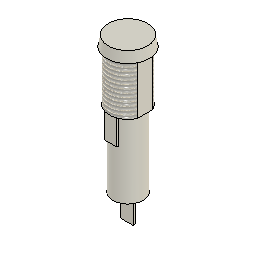
fuse holder 15A v2 (Autodesk Fusion 360 design; units mm, degrees)
Autodesk Fusion 360 part; units mm, degrees
note: some values were not read from the file. Set by a fixed rule: which face or edge a step refers to.
sketch "Sketch1" plane through (0, 0, 0) normal (0, 1, 0) x (1, 0, 0)
  line L0 (0, -54.2) -> (7.7947, -54.2)
  line L1 (7.7947, -54.2) -> (8.5, -50.2)
  line L2 (8.5, -50.2) -> (7.6, -50.2)
  line L3 (7.6, -50.2) -> (7.6, -30.2)
  line L4 (7.6, -30.2) -> (6, -30.2)
  line L5 (6, -30.2) -> (6, 0)
  line L6 (6, 0) -> (0, 0)
  line L7 (0, -54.2) -> (0, 0)
  dimension "d1" = 8.5
  dimension "d2" = 4
  dimension "d3" = 100
  dimension "d4" = 54.2
  dimension "d5" = 15.2
  dimension "d6" = 20
  dimension "d7" = 6
  constraint horizontal L0
  constraint parallel L0 L2
  constraint perpendicular L2 L3
  constraint perpendicular L3 L4
  constraint perpendicular L4 L5
  constraint perpendicular L5 L6
  constraint perpendicular L6 L7
  constraint coincident L6.end L7
  constraint coincident L6.end L7.end
  measures "d1" horizontal distance of L6.end L1.end
  measures "d2" vertical distance of L0.end L1.end
  measures "d3" angle of L0 L1
  measures "d4" vertical distance of L0.end L5.end
  measures "d6" distance of L2.end L3.end
  measures "d7" distance of L6.end L5
revolve "Revolve1" add sketch "Sketch1" angle 360 about axis through (0, 0, 54.2) along (0, 0, -1) makes body 1
sketch "Sketch2" plane through (0, 0, 30.2) normal (0, 0, -1) x (1, 0, 0)
  circle A0 centre (0, 0) radius 6
  circle A1 centre (0, 0) radius 7.6
  line L0 (-2.4, 6.8) -> (2.4, 6.8)
  line L1 (2.4, 6.8) -> (2.4, 6)
  line L2 (2.4, 6) -> (-2.4, 6)
  line L3 (-2.4, 6) -> (-2.4, 6.8)
  line L4 (0, 6.8) -> (0, 0) construction
  dimension "d9" = 4.8
  dimension "d10" = 0.8
  constraint horizontal L0
  constraint vertical L1
  constraint horizontal L2
  constraint vertical L3
  constraint midpoint L0 L4.start
  constraint coincident A0.centre A1.centre
  constraint vertical L4
  constraint tangent A0 L2
  measures "d9" distance of L0.start L0.end
  measures "d10" distance of L0.start L2.end
extrude "Extrude1" add sketch "Sketch2" along normal blind 10.2 separate body contours L0 L1 L2 L3 makes body 2
sketch "Sketch3" plane through (0, 0, 0) normal (0, 0, -1) x (1, 0, 0)
  circle A0 centre (0, 0) radius 6
  line L0 (-2.4, 0.4) -> (2.4, 0.4)
  line L1 (2.4, 0.4) -> (2.4, -0.4)
  line L2 (2.4, -0.4) -> (-2.4, -0.4)
  line L3 (-2.4, -0.4) -> (-2.4, 0.4)
  line L4 (2.4, 6) -> (2.4, 6.8)
  line L5 (-2.4, 6.8) -> (-2.4, 6)
  line L6 (2.4, 0.4) -> (-2.4, -0.4) construction
  constraint horizontal L0
  constraint vertical L1
  constraint horizontal L2
  constraint vertical L3
  constraint collinear L1 L4
  constraint collinear L3 L5
  constraint equal L3 L5
  constraint midpoint A0.centre L6
extrude "Extrude2" add sketch "Sketch3" along normal blind 10.2 contours L0 L1 L2 L3 bodies 1
sketch "Sketch4" plane through (0, 0, 30.2) normal (0, 0, -1) x (1, 0, 0)
  circle A0 centre (0, 0) radius 6
  circle A1 centre (0, 0) radius 7.6
  line L0 (6.8, -20) -> (-6.8, -20)
  line L1 (-6.8, -20) -> (-6.8, 20)
  line L2 (-6.8, 20) -> (6.8, 20)
  line L3 (6.8, 20) -> (6.8, -20)
  line L4 (6.8, -20) -> (-6.8, 20) construction
  line L5 (-6.8, -20) -> (6.8, 20) construction
  dimension "d15" = 13.6
  constraint horizontal L0
  constraint perpendicular L0 L1
  constraint parallel L0 L2
  constraint parallel L1 L3
  constraint coincident L4 A0.centre
  constraint coincident L5 A0.centre
  constraint coincident A0.centre A1.centre
  measures "d15" distance of L1.end L2.end
extrude "Extrude3" cut sketch "Sketch4" against normal blind 20 contours A1 L3 | A1 L1 bodies 1
thread "Thread1" "ISO Metric profile 15.0 M15x1.5 M15x1.5 6g" major diameter 14.85 minor diameter 13.1369 pitch 1.5 angle 60 resizes the face on face at (-6.4334, -4.0462, 43.5333) on face at (6.6247, 3.7247, 43.5333) on bodies 1
equation "d1 = ( 17 / 2 ) * 1 mm"
